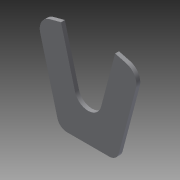
# Autodesk Inventor part: HW 6 Part 1
Saved by Autodesk Inventor 2015 SP1 (Build 190203100, 203)
## iProperties
Created: 2016-02-08
Part Number: HW 6 Part 1
Material: Generic
Document SubType Name: Modeling
Designer: melissa.roth
Density: 1 g/cm^3
Appearance: Default
Author: melissa.roth
Autodesk Inventor part; units mm, degrees
ref_plane "YZ Plane" through (0, 0, 0) normal (1, 0, 0) x (0, 1, 0)
ref_plane "XZ Plane" through (0, 0, 0) normal (0, 1, 0) x (-1, 0, 0)
ref_plane "XY Plane" through (0, 0, 0) normal (0, 0, 1) x (1, 0, 0)
sketch "Sketch1" plane through (0, 0, 0) normal (0, 0, 1) x (1, 0, 0)
  arc A0 (-50.7234, -1.9107) -> (-7.9329, -1.9107) centre (-29.3282, 3.7272) ccw
  line L0 (-7.9329, -1.9107) -> (15.0638, 85.3606)
  line L1 (15.0638, 85.3606) -> (33.485, 80.5064)
  line L2 (49.3132, 53.3519) -> (20.9478, -54.293)
  line L3 (5.5968, -66.1228) -> (-64.2532, -66.1228)
  line L4 (-79.6041, -54.293) -> (-107.9695, 53.3519)
  line L5 (-92.1413, 80.5064) -> (-73.7202, 85.3606)
  line L6 (-73.7202, 85.3606) -> (-50.7234, -1.9107)
  arc A1 (49.3132, 53.3519) -> (33.485, 80.5064) centre (27.8218, 59.0151) ccw
  arc A2 (-92.1413, 80.5064) -> (-107.9695, 53.3519) centre (-86.4782, 59.0151) ccw
  arc A3 (5.5968, -66.1228) -> (20.9478, -54.293) centre (5.5968, -50.2478) ccw
  arc A4 (-79.6041, -54.293) -> (-64.2532, -66.1228) centre (-64.2532, -50.2478) ccw
  dimension "d4" = 22.225
  dimension "d5" = 15.875
  dimension "d6" = 34.925
  dimension "d8" = 57.15
  dimension "d9" = 69.85
  dimension "d11" = 41.275
  dimension "d12" = 41.275
  constraints: 14 end point, 10 point on circle, 10 tangent, 5 centre point, 2 equal length, 2 equal radius, 2 parallel, 2 perpendicular, 1 horizontal
  measures "d4" radius of A1
  measures "d5" radius of A3
  measures "d6" horizontal distance of A0.centre L3.start
  measures "d8" horizontal distance of A1.centre A0.centre
  measures "d9" vertical distance of A0.centre L3.start
  measures "d11" distance between parallel lines of L2 L0
  measures "d12" distance between parallel lines of L4 L6
extrude "Extrusion1" add sketch "Sketch1" along normal blind 6.35
body "Solid1"
